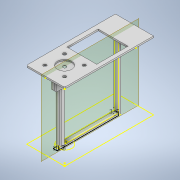
# Autodesk Inventor part: 42底座2
Saved by Autodesk Inventor 2022.5 (Build 265521000, 521)
## iProperties
Created: 2025-01-07
Part Number: 42底座2
Material: 常规
Document SubType Name: Modeling
Designer: Administrator
Density: 1 g/cm^3
Appearance: 默认
Mass: 23.3813 g
Surface Area: 205.342 cm^2
Volume: 23.3813 cm^3
Author: Administrator
Autodesk Inventor part; units mm, degrees
ref_plane "YZ Plane" through (0, 0, 0) normal (1, 0, 0) x (0, 1, 0)
ref_plane "XZ Plane" through (0, 0, 0) normal (0, 1, 0) x (-1, 0, 0)
ref_plane "XY Plane" through (0, 0, 0) normal (0, 0, 1) x (1, 0, 0)
sketch "草图1" plane through (0, 0, 0) normal (0, 1, 0) x (-1, 0, 0)
  line L0 (0, 0) -> (60, 0)
  line L1 (60, 0) -> (60, -140)
  line L2 (60, -140) -> (0, -140)
  line L3 (0, -140) -> (0, 0)
  dimension "d0" = 60
  dimension "d1" = 140
  constraints: 8 end point, 2 parallel, 1 horizontal, 1 perpendicular
  measures "d0" distance of L1.end L2.end
  measures "d1" distance of L0.end L1.end
extrude "拉伸1" add sketch "草图1" along normal blind 2.5
sketch "草图2" plane through (0, 2.5, 0) normal (0, 1, 0) x (1, 0, 0)
  line L0 (0, 140) -> (-60, 140) projected
  line L1 (-60, 140) -> (-60, 0) projected
  line L2 (-60, 0) -> (0, 0) projected
  line L3 (0, 0) -> (0, 140) projected
  line L4 (-60, 0) -> (0, 0) projected
  line L5 (-30, 0) -> (-30, 146.6003)
  line L6 (-30, 8.9185) -> (-51, 8.9185)
  line L7 (-51, 8.9185) -> (-51, 50.9185)
  line L8 (-51, 50.9185) -> (-30, 50.9185)
  line L9 (-30, 50.9185) -> (-30, 8.9185)
  line L10 (-30, 8.9185) -> (-9, 8.9185)
  line L11 (-9, 8.9185) -> (-9, 50.9185)
  line L12 (-9, 50.9185) -> (-30, 50.9185)
  circle A0 centre (-45.5, 14.4185) radius 2.9433
  line L13 (-51, 29.9185) -> (-35.5931, 29.9185)
  circle A1 centre (-45.5, 45.4185) radius 2.9433
  circle A2 centre (-14.5, 14.4185) radius 2.9433
  circle A3 centre (-14.5, 45.4185) radius 2.9433
  circle A4 centre (-30, 29.9185) radius 2.55
  circle A5 centre (-30, 29.9185) radius 11.25
  dimension "d4" = 21
  dimension "d5" = 42
  dimension "d6" = 31
  dimension "d7" = 31
  dimension "d12" = 5.1
  dimension "d15" = 22.5
  constraints: 18 end point, 6 centre point, 5 symmetric about line, 3 midpoint, 2 horizontal, 2 parallel, 1 coincident, 1 perpendicular, 1 point on line, 1 vertical, 3 other
  measures "d4" distance of L7.end L8.end
  measures "d5" distance of L6.end L7.end
  measures "d6" diameter of A0.centre L5
  measures "d7" diameter of A0.centre L13
  measures "d12" diameter of A4
  measures "d15" diameter of A5
extrude "拉伸4" cut sketch "草图2" along normal mid plane 10 contours A4 L5 | L5 A4
extrude "拉伸5" cut sketch "草图2" against normal blind 10 contours A5 L5 A4 | L5 A4 A5 | A4 L5 | L5 A4
extrude "拉伸6" cut sketch "草图2" against normal blind 10 contours A5 L5 A4 | L5 A4 A5 | A4 L5 | L5 A4
sketch "草图6" plane through (0, 0, 0) normal (0, -1, 0) x (1, 0, 0)
  line L0 (-9, -8.9185) -> (-51, -8.9185) projected
  circle A0 centre (-30, -29.9185) radius 2.55 projected
  line L1 (-30, -29.9185) -> (-26.8, -29.9185)
  line L2 (-26.8, -29.9185) -> (-26.8, -111.9185)
  line L3 (-30, -29.9185) -> (-30, -39.9264)
  line L4 (-30, -29.9185) -> (-33.2, -29.9185)
  line L5 (-33.2, -29.9185) -> (-33.2, -111.9185)
  line L6 (-26.8, -111.9185) -> (-31.6, -111.9185)
  line L7 (-31.6, -111.9185) -> (-33.2, -111.9185)
  line L8 (-26.8, -111.9185) -> (-33.2, -111.9185)
  line L9 (-33.2, -111.9185) -> (-33.2, -115.1185)
  line L10 (-33.2, -115.1185) -> (-26.8, -115.1185)
  line L11 (-26.8, -115.1185) -> (-26.8, -111.9185)
  point P0 (0, 0)
  dimension "d20" = 3.2
  dimension "d21" = 82
  dimension "d22" = 3.2
  constraints: 22 end point, 3 horizontal, 2 parallel, 2 perpendicular, 2 symmetric about line, 1 collinear, 1 vertical
  measures "d20" distance of L1.start L1.end
  measures "d21" distance of L1.end L2.end
  measures "d22" distance of L9.end L8.end
extrude "拉伸7" add sketch "草图6" along normal blind 105 contours L11 L10 L9 L7 L6
sketch "草图7" plane through (-33.2, 0, -111.9185) normal (0, 0, 1) x (1, 0, 0)
  line L0 (0, 0) -> (6.4, 0) projected
  line L1 (0, 0) -> (0, -105) projected
  line L2 (6.4, -105) -> (0, -105) projected
  line L3 (6.4, 0) -> (6.4, -105) projected
  line L4 (6.4, 0) -> (6.4, -105) projected
  line L5 (0, 0) -> (0, -105) projected
  line L6 (6.4, -105) -> (0, -105)
  line L7 (0, -105) -> (0, -101.5)
  line L8 (0, -101.5) -> (6.4, -101.5)
  line L9 (6.4, -101.5) -> (6.4, -105)
  point P0 (33.2, 0)
  dimension "d25" = 3.5
  constraints: 8 end point, 2 parallel, 1 horizontal, 1 perpendicular, 1 point on line
  measures "d25" distance of L6.end L7.end
sketch "草图8" plane through (0, -105, 0) normal (0, -1, 0) x (1, 0, 0)
  line L0 (-26.8, -111.9185) -> (-26.8, -115.1185) projected
  line L1 (-26.8, -115.1185) -> (-33.2, -115.1185) projected
  line L2 (-33.2, -115.1185) -> (-33.2, -111.9185) projected
  line L3 (-33.2, -111.9185) -> (-26.8, -111.9185) projected
  circle A0 centre (-30, -29.9185) radius 11.25 projected
  line L4 (0, -140) -> (-60, -140) projected
  line L5 (0, 0) -> (0, -140) projected
  line L6 (-60, 0) -> (0, 0) projected
  line L7 (-60, -140) -> (-60, 0) projected
  line L8 (-26.8, -111.9185) -> (-26.8, -29.9185)
  line L9 (-26.8, -29.9185) -> (-33.2, -29.9185)
  line L10 (-33.2, -29.9185) -> (-33.2, -111.9185)
  line L11 (-33.2, -111.9185) -> (-26.8, -111.9185)
  line L12 (-26.8, -111.9185) -> (-26.8, -29.9185)
  circle A1 centre (-30, -29.9185) radius 3.2
  line L13 (-26.8, -29.9185) -> (-26.8, -14.9185)
  line L14 (-26.8, -14.9185) -> (-33.2, -14.9185)
  line L15 (-33.2, -14.9185) -> (-33.2, -29.9185)
  circle A2 centre (-30, -29.9185) radius 2.55 projected
  line L16 (-26.8, -14.9185) -> (-26.8, -25.4185)
  line L17 (-26.8, -25.4185) -> (-33.2, -25.4185)
  dimension "d26" = 15
  dimension "d40" = 10.5
  constraints: 20 end point, 3 perpendicular, 3 vertical, 2 parallel, 2 point on line, 1 coincident, 1 collinear, 1 horizontal, 1 horizontal alignment, 2 other
  measures "d26" distance of L8.end L13.end
  measures "d40" distance of L13.end L16.end
extrude "拉伸8" add sketch "草图8" against normal blind 3.5 contours L3 L10 A0 L8 | A0 L10 A1 L8 | A1 L9 A2 | L9 A2 A1 | A1 L15 L17 L13 | L15 L14 L13 A0 | A0 L13 L17 L15
sketch "草图10" plane through (0, -105, 0) normal (0, -1, 0) x (1, 0, 0)
  line L0 (-26.8, -111.9185) -> (-26.8, -115.1185) projected
  line L1 (-26.8, -115.1185) -> (-33.2, -115.1185) projected
  line L2 (-33.2, -115.1185) -> (-33.2, -111.9185) projected
  line L3 (-33.2, -111.9185) -> (-26.8, -111.9185) projected
  circle A0 centre (-30, -29.9185) radius 11.25 projected
  line L4 (0, -140) -> (-60, -140) projected
  line L5 (0, 0) -> (0, -140) projected
  line L6 (-60, 0) -> (0, 0) projected
  line L7 (-60, -140) -> (-60, 0) projected
  circle A1 centre (-30, -29.9185) radius 2.55 projected
  line L8 (-33.2, -14.9185) -> (-33.2, -115.1185) projected
  line L9 (-33.2, -115.1185) -> (-26.8, -115.1185) projected
  line L10 (-26.8, -115.1185) -> (-26.8, -14.9185) projected
  line L11 (-26.8, -14.9185) -> (-33.2, -14.9185) projected
  circle A2 centre (-30, -29.9185) radius 3.05
  point P0 (-33.2, -19.1332)
  point P1 (-26.8, -19.1332)
  dimension "d31" = 6.1
  constraints: 1 centre point, 1 coincident
  measures "d31" diameter of A2
extrude "拉伸9" add sketch "草图10" against normal up to surface (105 mm away) contours A0 L8 L11 L10
extrude "拉伸10" cut sketch "草图10" against normal up to surface (3.5 mm away) contours A2
sketch "草图11" plane through (-33.2, -105, -115.1185) normal (-1, 0, 0) x (0, 0, 1)
  line L0 (3.2, 3.5) -> (95.9853, 3.5) projected
  line L1 (3.2, 105) -> (3.2, 3.5) projected
  line L2 (0, 105) -> (3.2, 105) projected
  line L3 (0, 105) -> (0, 0) projected
  line L4 (100.2, 0) -> (0, 0) projected
  line L5 (100.2, 0) -> (100.2, 105) projected
  line L6 (95.9853, 105) -> (100.2, 105) projected
  line L7 (95.9853, 3.5) -> (95.9853, 105) projected
  point P0 (115.1185, 105)
extrude "拉伸11" add sketch "草图11" along normal blind 1
sketch "草图12" plane through (0, 0, 0) normal (0, -1, 0) x (1, 0, 0)
  point P0 (0, 0)
extrude "拉伸12" add sketch "草图2" against normal up to surface (2.5 mm away) contours A5 L5 A4 | L5 A4 A5
sketch "草图13" plane through (-30, 2.5, -29.9185) normal (0, 1, 0) x (1, 0, 0)
  point P0 (30, -29.9185)
extrude "拉伸13" cut sketch "草图2" against normal blind 2 contours A5 L5 A4 | L5 A4 A5
sketch "草图14" plane through (0, -105, 0) normal (0, -1, 0) x (1, 0, 0)
  circle A0 centre (-30, -29.9185) radius 3.05 projected
  line L0 (-26.8, -115.1185) -> (-34.2, -115.1185) projected
  line L1 (-26.8, -14.9185) -> (-34.2, -14.9185) projected
  line L2 (-34.2, -115.1185) -> (-34.2, -14.9185) projected
  line L3 (-34.2, -115.1185) -> (-34.2, -14.9185) projected
  line L4 (-34.2, -19.1332) -> (-34.2, -14.9185) projected
  line L5 (-34.2, -19.1332) -> (-34.2, -111.9185) projected
  line L6 (-34.2, -115.1185) -> (-34.2, -111.9185) projected
  line L7 (-33.2, -19.1332) -> (-34.2, -19.1332) projected
  line L8 (-34.2, -19.1332) -> (-25.8, -19.1332)
  line L9 (-25.8, -115.1185) -> (-25.8, -14.9185) projected
  line L10 (-26.8, -115.1185) -> (-26.8, -14.9185) projected
  point P0 (0, 0)
  point P1 (-26.8, -19.1332)
  constraints: 2 end point, 1 horizontal, 1 point on line
extrude "拉伸14" cut sketch "草图14" against normal up to surface (105 mm away) contours L8 L7 L2 L1 L10
sketch "草图15" plane through (0, -101.5, 0) normal (0, 1, 0) x (1, 0, 0)
  line L0 (-34.2, 111.9185) -> (-26.8, 111.9185) projected
  line L1 (-34.2, 19.1332) -> (-34.2, 111.9185) projected
  circle A0 centre (-30, 29.9185) radius 3.05 projected
  line L2 (-26.8, 25.4185) -> (-33.2, 25.4185) projected
  line L3 (-26.8, 14.9185) -> (-26.8, 25.4185) projected
  line L4 (-34.2, 19.1332) -> (-26.8, 19.1332) projected
  line L5 (-26.8, 19.1332) -> (-26.8, 111.9185) projected
  point P0 (0, 0)
sketch "草图16" plane through (0, -105, 0) normal (0, -1, 0) x (1, 0, 0)
  line L0 (-26.8, -25.4185) -> (-33.2, -25.4185) projected
  line L1 (-34.2, -115.1185) -> (-34.2, -19.1332) projected
  line L2 (-26.8, -115.1185) -> (-34.2, -115.1185) projected
  circle A0 centre (-30, -29.9185) radius 3.05 projected
  line L3 (-26.8, -19.1332) -> (-34.2, -19.1332) projected
  line L4 (-26.8, -115.1185) -> (-26.8, -19.1332) projected
  point P0 (0, 0)
sketch "草图17" plane through (0, -101.5, 0) normal (0, 1, 0) x (1, 0, 0)
  line L0 (-25.8, 19.1332) -> (-34.2, 19.1332) projected
  line L1 (-25.8, 19.1332) -> (-25.8, 111.9185) projected
  line L2 (-34.2, 19.1332) -> (-25.8, 19.1332)
  line L3 (-25.8, 19.1332) -> (-25.8, 25.4182)
  line L4 (-25.8, 25.4182) -> (-34.2, 25.4182)
  line L5 (-34.2, 25.4182) -> (-34.2, 19.1332)
  point P0 (0, 0)
  dimension "d43" = 6.285
  constraints: 8 end point, 2 parallel, 1 horizontal, 1 perpendicular, 1 point on line
  measures "d43" distance of L3.end L2.end
extrude "拉伸15" add sketch "草图17" along normal up to surface (101.5 mm away)
fillet "圆角1" radius 2 3 edges at (-34.2, -52.5, -19.1332) (-25.8, -50.75, -19.1332) (-34.2, -52.5, -115.1185)
sketch "草图18" plane through (0, 2.5, 0) normal (0, 1, 0) x (1, 0, 0)
  circle A0 centre (-30, 29.9185) radius 11.25 projected
  line L0 (0, 140) -> (-60, 140) projected
  line L1 (-60, 140) -> (-60, 0) projected
  line L2 (-60, 0) -> (0, 0) projected
  line L3 (0, 0) -> (0, 140) projected
  circle A1 centre (-45.5, 14.4185) radius 2.5
  line L4 (-30, 29.9185) -> (-30, 12.6275)
  circle A2 centre (-45.5, 45.4185) radius 2.5
  point P0 (-14.5, 14.4185)
  dimension "d47" = 5
  dimension "d48" = 5
  constraints: 2 centre point, 2 coincident, 2 end point, 1 vertical
  measures "d47" diameter of A1
  measures "d48" diameter of A2
extrude "拉伸16" cut sketch "草图18" against normal blind 10 contours A1 | A2
ref_plane "工作平面2" through (-30, 0, -140) normal (-1, 0, 0) x (0, 0, 1)
mirror "镜像2" about plane through (-30, 0, -140) normal (-1, 0, 0) of "拉伸16"
sketch "草图19" plane through (0, 0, 0) normal (0, -1, 0) x (1, 0, 0)
  line L0 (0, -140) -> (-60, -140) projected
  line L1 (0, -140) -> (-110, -140)
  line L2 (-110, -140) -> (-110, -250)
  line L3 (-110, -250) -> (0, -250)
  line L4 (0, -250) -> (0, -140)
  circle A0 centre (-8, -146.46) radius 1.6
  circle A1 centre (-8, -242) radius 1.6
  circle A2 centre (-103.1, -146.46) radius 1.6
  circle A3 centre (-103.1, -242) radius 1.6
  point P0 (0, 0)
  dimension "d51" = 110
  dimension "d52" = 110
  dimension "d53" = 3.2
  dimension "d54" = 3.2
  dimension "d55" = 95.54
  dimension "d56" = 8
  dimension "d57" = 3.2
  dimension "d58" = 95.1
  dimension "d59" = 3.2
  dimension "d74" = 8
  dimension "d75" = 8
  dimension "d76" = 95.1
  constraints: 8 end point, 4 centre point, 2 parallel, 1 horizontal, 1 perpendicular
  measures "d51" distance of L2.end L1.end
  measures "d52" distance of L2.end L3.end
  measures "d53" diameter of A0
  measures "d54" diameter of A1
  measures "d55" distance of A1.centre A0.centre
  measures "d56" distance from line of L3 A1.centre
  measures "d57" diameter of A2
  measures "d58" distance of A0.centre A2.centre
  measures "d59" diameter of A3
  measures "d74" distance from line of L4 A0.centre
  measures "d75" distance from line of L4 A1.centre
  measures "d76" distance of A3.centre A1.centre
extrude "拉伸17" add sketch "草图19" against normal up to surface (2.5 mm away)
sketch "草图20" plane through (-25.8, -101.5, -25.4182) normal (1, 0, 0) x (0, 0, -1)
  line L0 (-4.285, 0) -> (-4.285, 101.5) projected
  line L1 (-4.285, 0) -> (0, 0) projected
  line L2 (0, 0) -> (0, 101.5) projected
  line L3 (-4.285, 101.5) -> (0, 101.5) projected
  line L4 (-4.285, 0) -> (-4.285, 101.5) projected
  line L5 (-4.285, 101.5) -> (-4.285, 85)
  line L6 (-4.285, 85) -> (0, 85)
  line L7 (0, 0) -> (0, 101.5) projected
  line L8 (-4.285, 85) -> (-8.285, 85)
  line L9 (-8.285, 85) -> (-8.285, 101.5)
  line L10 (114.5818, 101.5) -> (-25.4182, 101.5) projected
  line L11 (-6.285, 78.0536) -> (-14.0927, 78.0536)
  line L12 (-14.0927, 78.0536) -> (-14.0927, 101.5)
  line L13 (-6.285, 101.5) -> (-6.285, -3.5) projected
  point P0 (-6.285, 85)
  dimension "d62" = 16.5
  dimension "d63" = 4
  constraints: 12 end point, 4 point on line, 2 horizontal, 2 perpendicular, 1 vertical
  measures "d62" distance of L0.end L5.end
  measures "d63" distance of L5.end L8.end
extrude "拉伸18" cut sketch "草图20" along normal mid plane 20.75 contours L8 L13 L10 L0 | L0 L3 L2 L6 | L8 L9 L10 L13
extrude "拉伸19" add sketch "草图20" against normal blind 7.4 contours L13 L11 L12 L10 L9 L8
sketch "草图21" plane through (-25.8, -23.4464, -19.1332) normal (0, 0, -1) x (-1, 0, 0)
  line L0 (2, 6.9464) -> (2, 0) projected
  line L1 (0, 6.9464) -> (2, 6.9464) projected
  line L2 (0, 0) -> (0, 6.9464) projected
  line L3 (0, 0) -> (2, 0) projected
  line L4 (6.4, 0) -> (6.4, 6.9464) projected
  line L5 (6.4, 0) -> (7.4, 0) projected
  line L6 (7.4, 6.9464) -> (7.4, 0) projected
  line L7 (6.4, 6.9464) -> (7.4, 6.9464) projected
  point P0 (-25.8, 23.4464)
extrude "拉伸20" add sketch "草图21" along normal blind 2.5
fillet "圆角2" radius 2 3 edges at (-29.5, -23.4464, -11.3254) (-25.8, -11.7232, -11.3254) (-33.2, -11.7232, -11.3254)
sketch "草图22" plane through (0, -105, 0) normal (0, -1, 0) x (1, 0, 0)
  circle A0 centre (-30, -29.9185) radius 3.05 projected
  circle A1 centre (-30, -29.9185) radius 3.2 projected
  point P0 (0, 0)
sketch "草图23" plane through (0, -105, 0) normal (0, -1, 0) x (1, 0, 0)
  circle A0 centre (-30, -29.9185) radius 2.55 projected
  point P0 (0, 0)
sketch "草图24" plane through (0, -105, 0) normal (0, -1, 0) x (1, 0, 0)
  point P0 (0, 0)
sketch "草图25" plane through (0, -105, 0) normal (0, -1, 0) x (1, 0, 0)
  circle A0 centre (-30, -29.9185) radius 2.75
  point P0 (0, 0)
  dimension "d71" = 5.5
  constraints: 1 centre point, 1 coincident
  measures "d71" diameter of A0
extrude "拉伸21" cut sketch "草图25" against normal blind 2.5
sketch "草图26" plane through (0, 0, 0) normal (1, 0, 0) x (0, 0, -1)
  point P0 (0, 0)
sketch "草图27" plane through (0, 2.5, 0) normal (0, 1, 0) x (1, 0, 0)
  circle A0 centre (-8, 146.46) radius 1.6 projected
  circle A1 centre (-8, 242) radius 1.6 projected
  circle A2 centre (-103.1, 146.46) radius 1.6 projected
  circle A3 centre (-103.1, 242) radius 1.6 projected
  circle A4 centre (-14.5, 14.4185) radius 2.5 projected
  circle A5 centre (-14.5, 45.4185) radius 2.5 projected
  circle A6 centre (-45.5, 14.4185) radius 2.5 projected
  circle A7 centre (-45.5, 45.4185) radius 2.5 projected
  circle A8 centre (-30, 29.9185) radius 11.25 projected
  line L0 (-60, 140) -> (-60, 0) projected
  line L1 (-60, 0) -> (0, 0) projected
  line L2 (0, 0) -> (0, 250) projected
  line L3 (-110, 250) -> (0, 250) projected
  line L4 (-110, 140) -> (-110, 250) projected
  line L5 (-60, 140) -> (-110, 140) projected
  circle A9 centre (-8, 154.4212) radius 1.6
  circle A10 centre (-8, 234.4212) radius 1.6
  dimension "d77" = 3.2
  dimension "d78" = 3.2
  dimension "d79" = 80
  constraints: 2 centre point
  measures "d77" diameter of A9
  measures "d78" diameter of A10
  measures "d79" distance of A10.centre A9.centre
extrude "拉伸22" cut sketch "草图27" against normal up to surface (2.5 mm away) contours A9 | A10
sketch "草图28" plane through (0, 0, 0) normal (0, -1, 0) x (1, 0, 0)
  line L0 (-12.63, -150.06) -> (-99.8327, -150.06)
  line L1 (-99.8327, -150.06) -> (-99.8327, -239)
  line L2 (-99.8327, -239) -> (-12.63, -239)
  line L3 (-12.63, -239) -> (-12.63, -150.06)
  circle A0 centre (-8, -146.46) radius 1.6 projected
  circle A1 centre (-8, -242) radius 1.6 projected
  point P0 (0, 0)
  dimension "d82" = 3.6
  dimension "d83" = 3
  constraints: 8 end point, 2 parallel, 1 horizontal, 1 perpendicular
  measures "d82" distance from line of A0.centre L0
  measures "d83" distance from line of L2 A1.centre
extrude "拉伸23" cut sketch "草图28" against normal blind 10 contours L3 L2 L1 L0
fillet "圆角3" radius 2 5 edges at (-110, 1.25, -250) (0, 1.25, -250) (-110, 1.25, -140) (-60, 1.25, 0) (0, 1.25, 0)
sketch "草图29" plane through (0, 0, 0) normal (0, -1, 0) x (1, 0, 0)
  line L0 (-6, -56.5984) -> (-53, -56.5984)
  line L1 (-53, -56.5984) -> (-53, -105.9913)
  line L2 (-53, -105.9913) -> (-6, -105.9913)
  line L3 (-6, -105.9913) -> (-6, -56.5984)
  line L4 (-60, -140) -> (-60, -2) projected
  line L5 (0, -2) -> (0, -248) projected
  point P0 (0, 0)
  dimension "d87" = 7
  dimension "d88" = 6
  constraints: 8 end point, 2 parallel, 1 horizontal, 1 perpendicular
  measures "d87" distance between parallel lines of L4 L1
  measures "d88" distance between parallel lines of L5 L3
extrude "拉伸24" cut sketch "草图29" against normal blind 10
sketch "草图30" plane through (-30, 0, -140) normal (-1, 0, 0) x (0, 0, 1)
  point P0 (140, 0)
sketch "草图31" plane through (0, 0, 0) normal (0, -1, 0) x (1, 0, 0)
  line L0 (-6, -105.9913) -> (-53, -105.9913) projected
  line L1 (-53, -105.9913) -> (-53, -56.5984) projected
  line L2 (-53, -56.5984) -> (-6, -56.5984) projected
  line L3 (-6, -56.5984) -> (-6, -105.9913) projected
  circle A0 centre (-8, -146.46) radius 1.6 projected
  circle A1 centre (-8, -242) radius 1.6 projected
  circle A2 centre (-103.1, -146.46) radius 1.6 projected
  circle A3 centre (-103.1, -242) radius 1.6 projected
  circle A4 centre (-14.5, -14.4185) radius 2.5 projected
  circle A5 centre (-14.5, -45.4185) radius 2.5 projected
  circle A6 centre (-45.5, -14.4185) radius 2.5 projected
  circle A7 centre (-45.5, -45.4185) radius 2.5 projected
  circle A8 centre (-30, -29.9185) radius 2.55 projected
  arc A9 (0, -2) -> (-2, 0) centre (-2, -2) ccw projected
  line L4 (-58, 0) -> (-2, 0) projected
  arc A10 (-58, 0) -> (-60, -2) centre (-58, -2) ccw projected
  line L5 (-60, -140) -> (-60, -2) projected
  line L6 (-60, -140) -> (-108, -140) projected
  arc A11 (-108, -140) -> (-110, -142) centre (-108, -142) ccw projected
  line L7 (-110, -142) -> (-110, -248) projected
  arc A12 (-110, -248) -> (-108, -250) centre (-108, -248) ccw projected
  line L8 (-108, -250) -> (-2, -250) projected
  arc A13 (-2, -250) -> (0, -248) centre (-2, -248) ccw projected
  line L9 (0, -2) -> (0, -248) projected
  line L10 (-34.2, -111.9185) -> (-26.8, -111.9185) projected
  line L11 (-26.8, -111.9185) -> (-26.8, -115.1185) projected
  line L12 (-26.8, -115.1185) -> (-32.2, -115.1185) projected
  arc A14 (-34.2, -113.1185) -> (-32.2, -115.1185) centre (-32.2, -113.1185) ccw projected
  line L13 (-34.2, -113.1185) -> (-34.2, -111.9185) projected
  line L14 (-31.2, -11.3254) -> (-27.8, -11.3254) projected
  arc A15 (-25.8, -13.3254) -> (-27.8, -11.3254) centre (-27.8, -13.3254) ccw projected
  line L15 (-25.8, -13.3254) -> (-25.8, -17.1332) projected
  line L16 (-25.8, -17.1332) -> (-33.2, -17.1332) projected
  line L17 (-33.2, -17.1332) -> (-33.2, -13.3254) projected
  arc A16 (-31.2, -11.3254) -> (-33.2, -13.3254) centre (-31.2, -13.3254) ccw projected
  circle A17 centre (-8, -234.4212) radius 1.6 projected
  circle A18 centre (-8, -154.4212) radius 1.6 projected
  line L18 (-12.63, -239) -> (-99.8327, -239) projected
  line L19 (-99.8327, -239) -> (-99.8327, -150.06) projected
  line L20 (-99.8327, -150.06) -> (-12.63, -150.06) projected
  line L21 (-12.63, -150.06) -> (-12.63, -239) projected
  line L22 (0, -2) -> (0, -248) projected
  line L23 (-60, -140) -> (-60, -2) projected
  line L24 (0, -140) -> (-60, -140)
  point P0 (0, 0)
  constraints: 2 end point, 1 horizontal, 1 point on line
extrude "拉伸25" cut sketch "草图31" along normal blind 10 and the other way blind 5 contours L9 A13 L8 A12 L7 A11 L6 L24
sketch "草图32" plane through (-34.2, -105, -115.1185) normal (-1, 0, 0) x (0, 0, 1)
  line L0 (89.7003, 3.5) -> (3.2, 3.5) projected
  line L1 (89.7003, 3.5) -> (89.7003, 2)
  line L2 (89.7003, 2) -> (3.2, 2)
  line L3 (2, 0) -> (2, 105) projected
  line L4 (3.2, 105) -> (3.2, 3.5) projected
  line L5 (3.2, 2) -> (3.2, 3.5)
  point P0 (115.1185, 105)
  dimension "d95" = 1.5
  constraints: 6 end point, 2 perpendicular, 1 vertical
  measures "d95" distance between parallel lines of L0 L2
extrude "拉伸26" cut sketch "草图32" against normal blind 10
